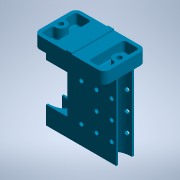
# Autodesk Inventor part: P108
Saved by Autodesk Inventor 2020 (Build 240168000, 168)
## iProperties
Created: 2016-10-19
Part Number: P108
Material: ABS Plastic
Document SubType Name: Modeling
Designer: serge.amoos
Density: 1.06 g/cm^3
Appearance: Sky Blue Medium
Mass: 20.1412 g
Surface Area: 89.2069 cm^2
Volume: 19.0012 cm^3
Description: Entretoise pour caméra
Author: serge.amoos
Autodesk Inventor part; units mm, degrees
ref_plane "YZ Plane" through (0, 0, 0) normal (1, 0, 0) x (0, 1, 0)
ref_plane "XZ Plane" through (0, 0, 0) normal (0, 1, 0) x (-1, 0, 0)
ref_plane "XY Plane" through (0, 0, 0) normal (0, 0, 1) x (1, 0, 0)
sketch "Sketch1" plane through (0, 0, 0) normal (0, 0, 1) x (1, 0, 0)
  line L0 (-36, 0) -> (6, 0) construction
  line L1 (0, -25.2) -> (0, 25.2) construction
  line L2 (-30, 18) -> (0, 18)
  line L3 (0, 18) -> (0, -18)
  line L4 (0, -18) -> (-30, -18)
  line L5 (-30, -18) -> (-30, 18)
  point P0 (0, 0)
  point P1 (0, 0)
  dimension "d0" = 36
  dimension "d1" = 30
  constraints: 8 end point, 2 parallel, 2 point on line, 1 horizontal, 1 midpoint, 1 perpendicular
  measures "d0" distance of L4.end L2.start
  measures "d1" distance of L2.start L2.end
extrude "Extrusion1" add sketch "Sketch1" along normal blind 10
sketch "Sketch2" plane through (0, 0, 10) normal (0, 0, 1) x (1, 0, 0)
  line L0 (-36, 0) -> (6, 0) construction
  line L1 (0, -25.2) -> (0, 25.2) construction
  point P0 (0, 0)
  point P1 (-25, 0)
  dimension "d5" = 25
  constraints: 1 point on line
  measures "d5" distance from line of L1 point (-25, 0)
hole "Hole1" at (-25, 0, 10) direction (0, 0, -1) diameter 4.2 end through all
fillet "Fillet1" radius 5 2 edges at (-30, -18, 5) (-30, 18, 5)
sketch "Sketch5" plane through (0, 0, 10) normal (0, 0, 1) x (1, 0, 0)
  line L0 (-14, 0) -> (-14, -15)
  line L1 (-14, -15) -> (-27, -15)
  line L2 (-27, -15) -> (-27, -5)
  line L3 (-27, -5) -> (-20, -5)
  line L4 (-20, -5) -> (-20, 0)
  line L5 (-20, 0) -> (-14, 0)
  line L6 (-25, -18) -> (0, -18) projected
  line L7 (-30, 13) -> (-30, -13) projected
  line L8 (-36, 0) -> (6, 0) projected
  line L9 (0, -18) -> (0, 18) projected
  point P0 (0, 0)
  dimension "d27" = 3
  dimension "d28" = 3
  dimension "d29" = 5
  dimension "d30" = 14
  dimension "d31" = 6
  constraints: 12 end point, 4 perpendicular, 1 collinear, 1 vertical
  measures "d27" distance between parallel lines of L6 L1
  measures "d28" distance between parallel lines of L7 L2
  measures "d29" distance between parallel lines of L8 L3
  measures "d30" distance between parallel lines of L9 L0
  measures "d31" distance between parallel lines of L0 L4
extrude "Extrusion3" cut sketch "Sketch5" against normal blind 9
fillet "Fillet2" radius 2 2 edges at (-27, -15, 5.5) (-14, -15, 5.5)
fillet "Fillet3" radius 2 1 edges at (-27, -5, 5.5)
fillet "Fillet4" radius 5 1 edges at (-20, -5, 5.5)
fillet "Fillet5" radius 1 9 edges at (-27, -10, 1) (-26.4142, -14.4142, 1) (-20.5, -15, 1) (-14.5858, -14.4142, 1) (-14, -6.5, 1) (-24.9999, -5, 1) (-21.4644, -3.5356, 1) (-20, 0, 1) (-26.4142, -5.5858, 1)
mirror "Mirror3" about plane through (-20, 0, 10) normal (0, -1, 0) of "Extrusion3", "Fillet2", "Fillet3", "Fillet4", "Fillet5"
mirror "Mirror2" about plane through (0, -18, 0) normal (1, 0, 0)
sketch "Sketch4" plane through (-30, -18, 0) normal (0, -1, 0) x (1, 0, 0)
  line L0 (5, 10) -> (55, 10) construction
  line L1 (30, -2.6) -> (30, 15.6) construction
  line L2 (27.5, 10) -> (32.5, 10)
  line L3 (32.5, 10) -> (32.5, 11)
  line L4 (32.5, 11) -> (27.5, 11)
  line L5 (27.5, 11) -> (27.5, 10)
  point P0 (30, 0)
  point P1 (0, 12)
  point P2 (60, 12)
  point P3 (30, 10)
  dimension "d22" = 1
  dimension "d23" = 5
  constraints: 8 end point, 2 parallel, 1 horizontal, 1 midpoint, 1 perpendicular, 1 point on line, 2 other
  measures "d23" distance of L3.end L4.end
extrude "Extrusion2" add sketch "Sketch4" against normal up to surface (36 mm away)
sketch "Sketch6" plane through (-30, -13, 0) normal (-1, 0, 0) x (0, 0, 1)
  line L0 (0, 20.5) -> (-64, 20.5)
  line L1 (-64, 20.5) -> (-64, 5.5)
  line L2 (-64, 5.5) -> (0, 5.5)
  line L3 (0, -5) -> (0, 0) projected
  line L4 (0, 0) -> (0, 26) projected
  line L5 (0, 26) -> (0, 31) projected
  dimension "d38" = 64
  dimension "d40" = 15
  dimension "d42" = 10.5
  dimension "d76" = 64
  constraints: 6 end point, 2 parallel, 1 horizontal, 1 point on line
  measures "d38" distance of L0.start L0.end
  measures "d40" distance of L0.end L1.end
  measures "d42" distance of L5.end L0.start
  measures "d76" distance of L1.end L2.end
extrude "Extrusion4" add sketch "Sketch6" against normal blind 60
sketch "Esquisse10" plane through (-30, -7.5, -64) normal (0, 0, -1) x (-1, 0, 0)
  line L0 (0, 0) -> (-60, 0) construction
  line L1 (0, 15) -> (-60, 15) construction
  line L2 (-30, -16.023) -> (-30, 37.6945) construction
  line L3 (0, 0) -> (0, 15) construction
  line L4 (-84.9535, 7.5) -> (17.8851, 7.5) construction
  ellipse E0 centre (0, 7.5) end of major axis (12, 7.5) minor radius 6
  line L5 (0, 15) -> (0, 0) construction
  line L6 (-60, 0) -> (-60, 15) construction
  ellipse E1 centre (-60, 7.5) end of major axis (-72, 7.5) minor radius 6
  line L7 (-60, 15) -> (-60, 0) construction
  point P0 (-30, 7.5)
  point P1 (-77.8851, 7.5)
  dimension "d58" = 12
  dimension "d59" = 6
  constraints: 10 end point, 8 symmetric about line, 3 point on line, 2 midpoint, 1 centre point, 1 horizontal, 1 vertical, 4 other
extrude "Extrusion5" cut sketch "Esquisse10" against normal up to surface (64 mm away)
sketch "Esquisse11" plane through (-30, 7.5, 0) normal (0, 1, 0) x (1, 0, 0)
  line L0 (5, -10) -> (27.5, -10) construction
  line L1 (95.7117, 32) -> (9.5422, 32) construction
  line L2 (95.7117, 16) -> (24.0518, 16) construction
  line L3 (60, 64) -> (60, 0) construction
  line L4 (43, 19.364) -> (43, 72.1681) construction
  line L5 (56, 17.0682) -> (56, 73.6604) construction
  line L6 (83.714, 48) -> (1.1498, 48) construction
  line L7 (30, 13.9903) -> (30, 74.2043) construction
  line L8 (0, 0) -> (0, 64) construction
  line L9 (0, 0) -> (5, 0) projected
  point P0 (30, 0)
  point P1 (56, 16)
  point P2 (30, 16)
  point P3 (30, 48)
  point P4 (56, 48)
  point P5 (43, 16)
  point P6 (43, 48)
  point P7 (43, 32)
  point P8 (56, 32)
  dimension "d62" = 16
  dimension "d63" = 13
  dimension "d65" = 17
  dimension "d66" = 16
  dimension "d67" = 13
  dimension "d87" = 32
  constraints: 16 point on line, 12 end point, 3 horizontal, 3 vertical
  measures "d62" distance between parallel lines of L1 L2
  measures "d63" distance of point (56, 32) point (43, 32)
  measures "d65" distance between parallel lines of L3 L4
  measures "d66" distance between parallel lines of L6 L1
  measures "d67" distance between parallel lines of L4 L7
  measures "d87" distance between parallel lines of L1 L9
hole "Perçage3" at (26, 7.5, -16) at (0, 7.5, -16) at (0, 7.5, -48) at (26, 7.5, -48) at (13, 7.5, -16) at (13, 7.5, -48) at (13, 7.5, -32) at (26, 7.5, -32) direction (0, -1, 0) diameter 3.5 end through all
sketch "Esquisse13" plane through (-30, 7.5, 0) normal (0, 1, 0) x (1, 0, 0)
  line L0 (0, 15.5) -> (18, 15.5)
  line L1 (18, 15.5) -> (18, 48.5)
  line L2 (18, 48.5) -> (0, 48.5)
  line L3 (0, 48.5) -> (0, 15.5)
  line L4 (0, 0) -> (0, 64) construction
  line L5 (5, -10) -> (27.5, -10) construction
  line L6 (60, 0) -> (0, 0) projected
  point P0 (30, 0)
  dimension "d82" = 33
  dimension "d83" = 18
  dimension "d88" = 15.5
  constraints: 8 end point, 2 parallel, 1 horizontal, 1 perpendicular, 1 point on line
  measures "d82" distance between parallel lines of L2 L0
  measures "d83" distance between parallel lines of L3 L1
  measures "d88" distance between parallel lines of L0 L6
extrude "Extrusion6" cut sketch "Esquisse13" against normal through all
equation "\"d28\" = d27"
body "Solid1"
